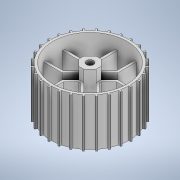
# Autodesk Inventor part: Reifen_v2
Saved by Autodesk Inventor 2021 (Build 250183000, 183)
## iProperties
Created: 2021-01-03
Part Number: Reifen_v2
Material: Generisch
Document SubType Name: Modeling
Designer: Ctroi
Density: 1 g/cm^3
Appearance: Vorgabe
Author: Ctroi
Autodesk Inventor part; units mm, degrees
ref_plane "YZ Plane" through (0, 0, 0) normal (1, 0, 0) x (0, 1, 0)
ref_plane "XZ Plane" through (0, 0, 0) normal (0, 1, 0) x (-1, 0, 0)
ref_plane "XY Plane" through (0, 0, 0) normal (0, 0, 1) x (1, 0, 0)
sketch "Skizze1" plane through (0, 0, 0) normal (0, 1, 0) x (-1, 0, 0)
  circle A0 centre (0, 0) radius 50
  circle A1 centre (0, 0) radius 47
  circle A2 centre (0, 0) radius 4.5
  line L0 (11, -3.1421) -> (3.1421, -11)
  line L1 (-3.1421, -11) -> (-11, -3.1421)
  line L2 (-11, 3.1421) -> (-3.1421, 11)
  line L3 (3.1421, 11) -> (11, 3.1421)
  line L4 (0, -70) -> (0, 70) projected
  line L5 (70, 0) -> (-70, 0) projected
  line L6 (3.1421, -11) -> (-3.1421, -11)
  line L7 (-11, -3.1421) -> (-11, 3.1421)
  line L8 (-3.1421, 11) -> (3.1421, 11)
  line L9 (11, 3.1421) -> (11, -3.1421)
  line L10 (3.1421, -11) -> (13.7487, -21.6066)
  line L11 (3.1421, -11) -> (18.1421, -11) construction
  line L12 (13.7487, -21.6066) -> (13.7487, -44.9441)
  line L13 (-3.1421, -11) -> (-13.7487, -21.6066)
  line L14 (-3.1421, -11) -> (11.8579, -11) construction
  line L15 (-13.7487, -21.6066) -> (-13.7487, -44.9441)
  line L16 (10.7487, -44.9441) -> (10.7487, -22.8492)
  line L17 (10.7487, -22.8492) -> (1.0208, -13.1213)
  line L18 (-10.7487, -44.9441) -> (-10.7487, -22.8492)
  line L19 (-10.7487, -22.8492) -> (-1.0208, -13.1213)
  line L20 (1.0208, -13.1213) -> (-1.0208, -13.1213)
  line L21 (10.7487, -44.9441) -> (10.7487, -45.7544)
  line L22 (-10.7487, -44.9441) -> (-10.7487, -45.7544)
  line L23 (21.6066, 13.7487) -> (44.9441, 13.7487)
  line L24 (44.9441, 10.7487) -> (22.8492, 10.7487)
  line L25 (44.9441, 10.7487) -> (45.7544, 10.7487)
  line L26 (44.9441, -10.7487) -> (45.7544, -10.7487)
  line L27 (44.9441, -10.7487) -> (22.8492, -10.7487)
  line L28 (21.6066, -13.7487) -> (44.9441, -13.7487)
  line L29 (22.8492, 10.7487) -> (13.1213, 1.0208)
  line L30 (11, 3.1421) -> (21.6066, 13.7487)
  line L31 (22.8492, -10.7487) -> (13.1213, -1.0208)
  line L32 (11, -3.1421) -> (21.6066, -13.7487)
  line L33 (13.1213, 1.0208) -> (13.1213, -1.0208)
  line L34 (-13.7487, 21.6066) -> (-13.7487, 44.9441)
  line L35 (-10.7487, 44.9441) -> (-10.7487, 22.8492)
  line L36 (-10.7487, 44.9441) -> (-10.7487, 45.7544)
  line L37 (10.7487, 44.9441) -> (10.7487, 45.7544)
  line L38 (10.7487, 44.9441) -> (10.7487, 22.8492)
  line L39 (13.7487, 21.6066) -> (13.7487, 44.9441)
  line L40 (-10.7487, 22.8492) -> (-1.0208, 13.1213)
  line L41 (-3.1421, 11) -> (-13.7487, 21.6066)
  line L42 (10.7487, 22.8492) -> (1.0208, 13.1213)
  line L43 (3.1421, 11) -> (13.7487, 21.6066)
  line L44 (-1.0208, 13.1213) -> (1.0208, 13.1213)
  line L45 (-21.6066, -13.7487) -> (-44.9441, -13.7487)
  line L46 (-44.9441, -10.7487) -> (-22.8492, -10.7487)
  line L47 (-44.9441, -10.7487) -> (-45.7544, -10.7487)
  line L48 (-44.9441, 10.7487) -> (-45.7544, 10.7487)
  line L49 (-44.9441, 10.7487) -> (-22.8492, 10.7487)
  line L50 (-21.6066, 13.7487) -> (-44.9441, 13.7487)
  line L51 (-22.8492, -10.7487) -> (-13.1213, -1.0208)
  line L52 (-11, -3.1421) -> (-21.6066, -13.7487)
  line L53 (-22.8492, 10.7487) -> (-13.1213, 1.0208)
  line L54 (-11, 3.1421) -> (-21.6066, 13.7487)
  line L55 (-13.1213, -1.0208) -> (-13.1213, 1.0208)
  dimension "d0" = 100
  dimension "d1" = 3
  dimension "d2" = 9
  dimension "d7" = 15
  dimension "d8" = 45
  dimension "d9" = 15
  dimension "d10" = 135
  dimension "d11" = 3
  dimension "d12" = 3
  dimension "d15" = 360
  constraints: 108 end point, 4 horizontal, 4 parallel, 4 point on circle, 4 vertical, 3 centre point, 2 coincident, 2 equal length, 2 perpendicular, 105 other
  measures "d0" diameter of A0
  measures "d1" radial gap between concentric circles of A0 A1
  measures "d2" diameter of A2
  measures "d7" distance of L0.end L10.end
  measures "d8" angle of L10 L11
  measures "d9" distance of L1.start L13.end
  measures "d10" angle of L13 L14
  measures "d11" distance between parallel lines of L12 L16
  measures "d12" distance between parallel lines of L15 L18
extrude "Extrusion1" add sketch "Skizze1" along normal blind 45 and the other way blind 15 contours L5 A1 L4 A0 | A0 L4 A1 L5 | L4 A1 L5 A0 | A0 L5 A1 L4
extrude "Extrusion2" add sketch "Skizze1" along normal blind 45 contours L9 L0 L6 L4 A2 L5 | L5 A2 L4 L8 L3 L9 | L4 A2 L5 L7 L2 L8 | L6 L1 L7 L5 A2 L4
extrude "Extrusion3" add sketch "Skizze1" along normal blind 30 contours L25 L24 L29 L33 L5 L9 L30 L23 A1 | A1 L28 L32 L9 L5 L33 L31 L27 L26 | A1 L39 L43 L8 L4 L44 L42 L38 L37 | L36 L35 L40 L44 L4 L8 L41 L34 A1 | A1 L15 L13 L6 L4 L20 L19 L18 L22 | L21 L16 L17 L20 L4 L6 L10 L12 A1 | A1 L50 L54 L7 L5 L55 L53 L49 L48 | L47 L46 L51 L55 L5 L7 L52 L45 A1
sketch "Skizze2" plane through (0, 45, 0) normal (0, 1, 0) x (1, 0, 0)
  circle A0 centre (0, 0) radius 50 projected
  line L0 (1, 49.99) -> (1, 52.49)
  line L1 (0.5, 52.99) -> (-0.5, 52.99)
  line L2 (-1, 52.49) -> (-1, 49.99)
  line L3 (0, 73.6) -> (0, -70.6) projected
  arc A1 (1, 52.49) -> (0.5, 52.99) centre (0.5, 52.49) ccw
  arc A2 (-0.5, 52.99) -> (-1, 52.49) centre (-0.5, 52.49) ccw
  line L4 (-10.1489, 48.9592) -> (-10.7052, 51.3965)
  arc A3 (-10.7052, 51.3965) -> (-11.3039, 51.7727) centre (-11.1927, 51.2852) ccw
  line L5 (-11.3039, 51.7727) -> (-12.2788, 51.5502)
  arc A4 (-12.2788, 51.5502) -> (-12.6551, 50.9514) centre (-12.1676, 51.0627) ccw
  line L6 (-12.6551, 50.9514) -> (-12.0987, 48.5141)
  line L7 (-20.7889, 45.4733) -> (-21.8736, 47.7257)
  arc A5 (-21.8736, 47.7257) -> (-22.541, 47.9593) centre (-22.3241, 47.5088) ccw
  line L8 (-22.541, 47.9593) -> (-23.442, 47.5254)
  arc A6 (-23.442, 47.5254) -> (-23.6755, 46.858) centre (-23.225, 47.0749) ccw
  line L9 (-23.6755, 46.858) -> (-22.5908, 44.6055)
  line L10 (-30.3864, 39.7072) -> (-31.9451, 41.6618)
  arc A7 (-31.9451, 41.6618) -> (-32.6478, 41.741) centre (-32.3361, 41.3501) ccw
  line L11 (-32.6478, 41.741) -> (-33.4296, 41.1175)
  arc A8 (-33.4296, 41.1175) -> (-33.5088, 40.4148) centre (-33.1179, 40.7266) ccw
  line L12 (-33.5088, 40.4148) -> (-31.9501, 38.4603)
  line L13 (-38.4603, 31.9501) -> (-40.4148, 33.5088)
  arc A9 (-40.4148, 33.5088) -> (-41.1175, 33.4296) centre (-40.7266, 33.1179) ccw
  line L14 (-41.1175, 33.4296) -> (-41.741, 32.6478)
  arc A10 (-41.741, 32.6478) -> (-41.6618, 31.9451) centre (-41.3501, 32.3361) ccw
  line L15 (-41.6618, 31.9451) -> (-39.7072, 30.3864)
  line L16 (-44.6055, 22.5908) -> (-46.858, 23.6755)
  arc A11 (-46.858, 23.6755) -> (-47.5254, 23.442) centre (-47.0749, 23.225) ccw
  line L17 (-47.5254, 23.442) -> (-47.9593, 22.541)
  arc A12 (-47.9593, 22.541) -> (-47.7257, 21.8736) centre (-47.5088, 22.3241) ccw
  line L18 (-47.7257, 21.8736) -> (-45.4733, 20.7889)
  line L19 (-48.5141, 12.0987) -> (-50.9514, 12.6551)
  arc A13 (-50.9514, 12.6551) -> (-51.5502, 12.2788) centre (-51.0627, 12.1676) ccw
  line L20 (-51.5502, 12.2788) -> (-51.7727, 11.3039)
  arc A14 (-51.7727, 11.3039) -> (-51.3965, 10.7052) centre (-51.2852, 11.1927) ccw
  line L21 (-51.3965, 10.7052) -> (-48.9592, 10.1489)
  line L22 (-49.99, 1) -> (-52.49, 1)
  arc A15 (-52.49, 1) -> (-52.99, 0.5) centre (-52.49, 0.5) ccw
  line L23 (-52.99, 0.5) -> (-52.99, -0.5)
  arc A16 (-52.99, -0.5) -> (-52.49, -1) centre (-52.49, -0.5) ccw
  line L24 (-52.49, -1) -> (-49.99, -1)
  line L25 (-48.9592, -10.1489) -> (-51.3965, -10.7052)
  arc A17 (-51.3965, -10.7052) -> (-51.7727, -11.3039) centre (-51.2852, -11.1927) ccw
  line L26 (-51.7727, -11.3039) -> (-51.5502, -12.2788)
  arc A18 (-51.5502, -12.2788) -> (-50.9514, -12.6551) centre (-51.0627, -12.1676) ccw
  line L27 (-50.9514, -12.6551) -> (-48.5141, -12.0987)
  line L28 (-45.4733, -20.7889) -> (-47.7257, -21.8736)
  arc A19 (-47.7257, -21.8736) -> (-47.9593, -22.541) centre (-47.5088, -22.3241) ccw
  line L29 (-47.9593, -22.541) -> (-47.5254, -23.442)
  arc A20 (-47.5254, -23.442) -> (-46.858, -23.6755) centre (-47.0749, -23.225) ccw
  line L30 (-46.858, -23.6755) -> (-44.6055, -22.5908)
  line L31 (-39.7072, -30.3864) -> (-41.6618, -31.9451)
  arc A21 (-41.6618, -31.9451) -> (-41.741, -32.6478) centre (-41.3501, -32.3361) ccw
  line L32 (-41.741, -32.6478) -> (-41.1175, -33.4296)
  arc A22 (-41.1175, -33.4296) -> (-40.4148, -33.5088) centre (-40.7266, -33.1179) ccw
  line L33 (-40.4148, -33.5088) -> (-38.4603, -31.9501)
  line L34 (-31.9501, -38.4603) -> (-33.5088, -40.4148)
  arc A23 (-33.5088, -40.4148) -> (-33.4296, -41.1175) centre (-33.1179, -40.7266) ccw
  line L35 (-33.4296, -41.1175) -> (-32.6478, -41.741)
  arc A24 (-32.6478, -41.741) -> (-31.9451, -41.6618) centre (-32.3361, -41.3501) ccw
  line L36 (-31.9451, -41.6618) -> (-30.3864, -39.7072)
  line L37 (-22.5908, -44.6055) -> (-23.6755, -46.858)
  arc A25 (-23.6755, -46.858) -> (-23.442, -47.5254) centre (-23.225, -47.0749) ccw
  line L38 (-23.442, -47.5254) -> (-22.541, -47.9593)
  arc A26 (-22.541, -47.9593) -> (-21.8736, -47.7257) centre (-22.3241, -47.5088) ccw
  line L39 (-21.8736, -47.7257) -> (-20.7889, -45.4733)
  line L40 (-12.0987, -48.5141) -> (-12.6551, -50.9514)
  arc A27 (-12.6551, -50.9514) -> (-12.2788, -51.5502) centre (-12.1676, -51.0627) ccw
  line L41 (-12.2788, -51.5502) -> (-11.3039, -51.7727)
  arc A28 (-11.3039, -51.7727) -> (-10.7052, -51.3965) centre (-11.1927, -51.2852) ccw
  line L42 (-10.7052, -51.3965) -> (-10.1489, -48.9592)
  line L43 (-1, -49.99) -> (-1, -52.49)
  arc A29 (-1, -52.49) -> (-0.5, -52.99) centre (-0.5, -52.49) ccw
  line L44 (-0.5, -52.99) -> (0.5, -52.99)
  arc A30 (0.5, -52.99) -> (1, -52.49) centre (0.5, -52.49) ccw
  line L45 (1, -52.49) -> (1, -49.99)
  line L46 (10.1489, -48.9592) -> (10.7052, -51.3965)
  arc A31 (10.7052, -51.3965) -> (11.3039, -51.7727) centre (11.1927, -51.2852) ccw
  line L47 (11.3039, -51.7727) -> (12.2788, -51.5502)
  arc A32 (12.2788, -51.5502) -> (12.6551, -50.9514) centre (12.1676, -51.0627) ccw
  line L48 (12.6551, -50.9514) -> (12.0987, -48.5141)
  line L49 (20.7889, -45.4733) -> (21.8736, -47.7257)
  arc A33 (21.8736, -47.7257) -> (22.541, -47.9593) centre (22.3241, -47.5088) ccw
  line L50 (22.541, -47.9593) -> (23.442, -47.5254)
  arc A34 (23.442, -47.5254) -> (23.6755, -46.858) centre (23.225, -47.0749) ccw
  line L51 (23.6755, -46.858) -> (22.5908, -44.6055)
  line L52 (30.3864, -39.7072) -> (31.9451, -41.6618)
  arc A35 (31.9451, -41.6618) -> (32.6478, -41.741) centre (32.3361, -41.3501) ccw
  line L53 (32.6478, -41.741) -> (33.4296, -41.1175)
  arc A36 (33.4296, -41.1175) -> (33.5088, -40.4148) centre (33.1179, -40.7266) ccw
  line L54 (33.5088, -40.4148) -> (31.9501, -38.4603)
  line L55 (38.4603, -31.9501) -> (40.4148, -33.5088)
  arc A37 (40.4148, -33.5088) -> (41.1175, -33.4296) centre (40.7266, -33.1179) ccw
  line L56 (41.1175, -33.4296) -> (41.741, -32.6478)
  arc A38 (41.741, -32.6478) -> (41.6618, -31.9451) centre (41.3501, -32.3361) ccw
  line L57 (41.6618, -31.9451) -> (39.7072, -30.3864)
  line L58 (44.6055, -22.5908) -> (46.858, -23.6755)
  arc A39 (46.858, -23.6755) -> (47.5254, -23.442) centre (47.0749, -23.225) ccw
  line L59 (47.5254, -23.442) -> (47.9593, -22.541)
  arc A40 (47.9593, -22.541) -> (47.7257, -21.8736) centre (47.5088, -22.3241) ccw
  line L60 (47.7257, -21.8736) -> (45.4733, -20.7889)
  line L61 (48.5141, -12.0987) -> (50.9514, -12.6551)
  arc A41 (50.9514, -12.6551) -> (51.5502, -12.2788) centre (51.0627, -12.1676) ccw
  line L62 (51.5502, -12.2788) -> (51.7727, -11.3039)
  arc A42 (51.7727, -11.3039) -> (51.3965, -10.7052) centre (51.2852, -11.1927) ccw
  line L63 (51.3965, -10.7052) -> (48.9592, -10.1489)
  line L64 (49.99, -1) -> (52.49, -1)
  arc A43 (52.49, -1) -> (52.99, -0.5) centre (52.49, -0.5) ccw
  line L65 (52.99, -0.5) -> (52.99, 0.5)
  arc A44 (52.99, 0.5) -> (52.49, 1) centre (52.49, 0.5) ccw
  line L66 (52.49, 1) -> (49.99, 1)
  line L67 (48.9592, 10.1489) -> (51.3965, 10.7052)
  arc A45 (51.3965, 10.7052) -> (51.7727, 11.3039) centre (51.2852, 11.1927) ccw
  line L68 (51.7727, 11.3039) -> (51.5502, 12.2788)
  arc A46 (51.5502, 12.2788) -> (50.9514, 12.6551) centre (51.0627, 12.1676) ccw
  line L69 (50.9514, 12.6551) -> (48.5141, 12.0987)
  line L70 (45.4733, 20.7889) -> (47.7257, 21.8736)
  arc A47 (47.7257, 21.8736) -> (47.9593, 22.541) centre (47.5088, 22.3241) ccw
  line L71 (47.9593, 22.541) -> (47.5254, 23.442)
  arc A48 (47.5254, 23.442) -> (46.858, 23.6755) centre (47.0749, 23.225) ccw
  line L72 (46.858, 23.6755) -> (44.6055, 22.5908)
  line L73 (39.7072, 30.3864) -> (41.6618, 31.9451)
  arc A49 (41.6618, 31.9451) -> (41.741, 32.6478) centre (41.3501, 32.3361) ccw
  line L74 (41.741, 32.6478) -> (41.1175, 33.4296)
  arc A50 (41.1175, 33.4296) -> (40.4148, 33.5088) centre (40.7266, 33.1179) ccw
  line L75 (40.4148, 33.5088) -> (38.4603, 31.9501)
  line L76 (31.9501, 38.4603) -> (33.5088, 40.4148)
  arc A51 (33.5088, 40.4148) -> (33.4296, 41.1175) centre (33.1179, 40.7266) ccw
  line L77 (33.4296, 41.1175) -> (32.6478, 41.741)
  arc A52 (32.6478, 41.741) -> (31.9451, 41.6618) centre (32.3361, 41.3501) ccw
  line L78 (31.9451, 41.6618) -> (30.3864, 39.7072)
  line L79 (22.5908, 44.6055) -> (23.6755, 46.858)
  arc A53 (23.6755, 46.858) -> (23.442, 47.5254) centre (23.225, 47.0749) ccw
  line L80 (23.442, 47.5254) -> (22.541, 47.9593)
  arc A54 (22.541, 47.9593) -> (21.8736, 47.7257) centre (22.3241, 47.5088) ccw
  line L81 (21.8736, 47.7257) -> (20.7889, 45.4733)
  line L82 (12.0987, 48.5141) -> (12.6551, 50.9514)
  arc A55 (12.6551, 50.9514) -> (12.2788, 51.5502) centre (12.1676, 51.0627) ccw
  line L83 (12.2788, 51.5502) -> (11.3039, 51.7727)
  arc A56 (11.3039, 51.7727) -> (10.7052, 51.3965) centre (11.1927, 51.2852) ccw
  line L84 (10.7052, 51.3965) -> (10.1489, 48.9592)
  point P0 (1, 52.99)
  point P1 (-1, 52.99)
  point P2 (-10.8165, 51.884)
  point P3 (-12.7663, 51.4389)
  point P4 (-22.0905, 48.1762)
  point P5 (-23.8925, 47.3085)
  point P6 (-32.2569, 42.0527)
  point P7 (-33.8206, 40.8058)
  point P8 (-40.8058, 33.8206)
  point P9 (-42.0527, 32.2569)
  point P10 (-47.3085, 23.8925)
  point P11 (-48.1762, 22.0905)
  point P12 (-51.4389, 12.7663)
  point P13 (-51.884, 10.8165)
  point P14 (-52.99, 1)
  point P15 (-52.99, -1)
  point P16 (-51.884, -10.8165)
  point P17 (-51.4389, -12.7663)
  point P18 (-48.1762, -22.0905)
  point P19 (-47.3085, -23.8925)
  point P20 (-42.0527, -32.2569)
  point P21 (-40.8058, -33.8206)
  point P22 (-33.8206, -40.8058)
  point P23 (-32.2569, -42.0527)
  point P24 (-23.8925, -47.3085)
  point P25 (-22.0905, -48.1762)
  point P26 (-12.7663, -51.4389)
  point P27 (-10.8165, -51.884)
  point P28 (-1, -52.99)
  point P29 (1, -52.99)
  point P30 (10.8165, -51.884)
  point P31 (12.7663, -51.4389)
  point P32 (22.0905, -48.1762)
  point P33 (23.8925, -47.3085)
  point P34 (32.2569, -42.0527)
  point P35 (33.8206, -40.8058)
  point P36 (40.8058, -33.8206)
  point P37 (42.0527, -32.2569)
  point P38 (47.3085, -23.8925)
  point P39 (48.1762, -22.0905)
  point P40 (51.4389, -12.7663)
  point P41 (51.884, -10.8165)
  point P42 (52.99, -1)
  point P43 (52.99, 1)
  point P44 (51.884, 10.8165)
  point P45 (51.4389, 12.7663)
  point P46 (48.1762, 22.0905)
  point P47 (47.3085, 23.8925)
  point P48 (42.0527, 32.2569)
  point P49 (40.8058, 33.8206)
  point P50 (33.8206, 40.8058)
  point P51 (32.2569, 42.0527)
  point P52 (23.8925, 47.3085)
  point P53 (22.0905, 48.1762)
  point P54 (12.7663, 51.4389)
  point P55 (10.8165, 51.884)
  dimension "d25" = 2
  dimension "d26" = 3
  dimension "d27" = 0.5
  dimension "d32" = 360
  constraints: 168 end point, 112 point on circle, 112 point on line, 56 centre point, 4 tangent, 2 parallel, 1 equal radius, 424 other
  measures "d25" distance of point (-1, 52.99) point (1, 52.99)
  measures "d26" distance of point (1, 52.99) L0.start
  measures "d27" radius of A1
extrude "Extrusion4" add sketch "Skizze2" against normal blind 60 contours A0 L3 L1 A1 L0 | A0 L2 A2 L1 L3
extrude "Extrusion5" add sketch "Skizze2" against normal blind 60 contours A0 L66 A44 L65 A43 L64 | A0 L69 A46 L68 A45 L67 | L63 A42 L62 A41 L61 A0 | A0 L72 A48 L71 A47 L70 | L60 A40 L59 A39 L58 A0 | A0 L75 A50 L74 A49 L73 | L57 A38 L56 A37 L55 A0 | A0 L78 A52 L77 A51 L76 | L54 A36 L53 A35 L52 A0 | A0 L81 A54 L80 A53 L79 | L51 A34 L50 A33 L49 A0 | A0 L84 A56 L83 A55 L82 | L48 A32 L47 A31 L46 A0 | L45 A30 L44 L3 A0 | L3 L44 A29 L43 A0 | A0 L6 A4 L5 A3 L4 | L42 A28 L41 A27 L40 A0 | A0 L9 A6 L8 A5 L7 | L39 A26 L38 A25 L37 A0 | A0 L12 A8 L11 A7 L10 | L36 A24 L35 A23 L34 A0 | A0 L15 A10 L14 A9 L13 | L33 A22 L32 A21 L31 A0 | A0 L18 A12 L17 A11 L16 | L30 A20 L29 A19 L28 A0 | A0 L21 A14 L20 A13 L19 | L27 A18 L26 A17 L25 A0 | A0 L24 A16 L23 A15 L22
